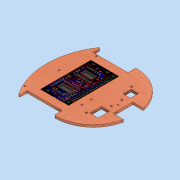
# Autodesk Inventor part: Version Raspberrry Pi Zero W
Saved by Autodesk Inventor 2022 (Build 260153000, 153)
## iProperties
Created: 2021-09-27
Part Number: Version Raspberrry Pi Zero W
Material: Madera (nogal)
Document SubType Name: Modeling
Designer: Julio R
Density: 0.55 g/cm^3
Appearance: Nogal - Natural pulido
Author: Julio R
Autodesk Inventor part; units mm, degrees
ref_plane "YZ Plane" through (0, 0, 0) normal (1, 0, 0) x (0, 1, 0)
ref_plane "XZ Plane" through (0, 0, 0) normal (0, 1, 0) x (-1, 0, 0)
ref_plane "XY Plane" through (0, 0, 0) normal (0, 0, 1) x (1, 0, 0)
sketch "Boceto2" plane through (0, 0, 0) normal (0, 1, 0) x (-1, 0, 0)
  circle A0 centre (-10.65, 0) radius 62.5
  line L0 (-44, 29.7) -> (-44, -29.3)
  line L1 (-41, -32.3) -> (-17, -32.3)
  line L2 (-14, -29.3) -> (-14, 29.7)
  line L3 (-17, 32.7) -> (-41, 32.7)
  circle A1 centre (-40.5, -28.8) radius 1.25
  line L4 (0, 6.809) -> (0, -6.809)
  line L5 (10.65, 0) -> (-10.65, 0) construction
  circle A2 centre (-17.5, -28.8) radius 1.25
  circle A3 centre (-40.5, 29.2) radius 1.25
  circle A4 centre (-17.5, 29.2) radius 1.25
  line L6 (7.5, -42.3) -> (-7, -42.3)
  line L7 (-7, -42.3) -> (-7, -25)
  line L8 (-7, -25) -> (7.5, -25)
  line L9 (7.5, -25) -> (7.5, -42.3)
  arc A5 (9.0958, -33.5419) -> (9.0958, -25.0441) centre (9, -29.293) ccw
  line L10 (9.0958, -33.5419) -> (7.5, -42.3)
  line L11 (9.0958, -25.0441) -> (7.5, -25.0441)
  arc A6 (9.5, -30.443) -> (9.5, -28.143) centre (9.5, -29.293) ccw
  line L12 (9.5, -30.443) -> (7.5, -30.443)
  line L13 (7.5, -30.443) -> (7.5, -28.143)
  line L14 (7.5, -28.143) -> (9.5, -28.143)
  line L15 (9.5, -28.143) -> (9.5, -30.443)
  arc A7 (-9.0958, -25.0441) -> (-9.0958, -33.5419) centre (-9, -29.293) ccw
  line L16 (-9.0958, -33.5419) -> (-7, -42.3)
  line L17 (-9.0958, -25.0441) -> (-7.5, -25.0441)
  arc A8 (-9.5, -28.143) -> (-9.5, -30.443) centre (-9.5, -29.293) ccw
  line L18 (-9.5, -30.443) -> (-7.5, -30.443)
  line L19 (-7.5, -30.443) -> (-7.5, -28.143)
  line L20 (-7.5, -28.143) -> (-9.5, -28.143)
  line L21 (-9.5, -28.143) -> (-9.5, -30.443)
  line L22 (7.5, 42.3) -> (-7, 42.3)
  line L23 (-7, 42.3) -> (-7, 25)
  line L24 (-7, 25) -> (7.5, 25)
  line L25 (7.5, 25) -> (7.5, 42.3)
  arc A9 (9.0958, 25.0441) -> (9.0958, 33.5419) centre (9, 29.293) ccw
  line L26 (9.0958, 33.5419) -> (7.5, 42.3)
  line L27 (9.0958, 25.0441) -> (7.5, 25.0441)
  arc A10 (9.5, 28.143) -> (9.5, 30.443) centre (9.5, 29.293) ccw
  line L28 (9.5, 30.443) -> (7.5, 30.443)
  line L29 (7.5, 30.443) -> (7.5, 28.143)
  line L30 (7.5, 28.143) -> (9.5, 28.143)
  line L31 (9.5, 28.143) -> (9.5, 30.443)
  line L32 (-9.0958, 25.0441) -> (-7.5, 25.0441)
  line L33 (-7.5, 28.143) -> (-9.5, 28.143)
  line L34 (-7.5, 30.443) -> (-7.5, 28.143)
  line L35 (-9.5, 28.143) -> (-9.5, 30.443)
  line L36 (-9.5, 30.443) -> (-7.5, 30.443)
  arc A11 (-9.5, 30.443) -> (-9.5, 28.143) centre (-9.5, 29.293) ccw
  line L37 (-9.0958, 33.5419) -> (-7, 42.3)
  arc A12 (-9.0958, 33.5419) -> (-9.0958, 25.0441) centre (-9, 29.293) ccw
  line L38 (10.3604, -4.25) -> (-9.8396, -4.25)
  line L39 (-9.8396, -4.25) -> (-9.8396, 4.25)
  line L40 (-9.8396, 4.25) -> (10.3604, 4.25)
  line L41 (10.3604, 4.25) -> (10.3604, -4.25)
  line L42 (35.3604, -42.3) -> (-56.6604, -42.3)
  line L43 (-56.6604, -42.3) -> (-56.6604, 42.3)
  line L44 (-56.6604, 42.3) -> (35.3604, 42.3)
  line L45 (35.3604, 42.3) -> (35.3604, -42.3)
  line L46 (-58.455, -12.75) -> (-68.455, -12.75)
  line L47 (-68.455, -12.75) -> (-68.455, 12.75)
  line L48 (-68.455, 12.75) -> (-58.455, 12.75)
  line L49 (-58.455, 12.75) -> (-58.455, -12.75)
  line L50 (22.5, 52.3) -> (-22.5, 52.3)
  line L51 (-22.5, 52.3) -> (-22.5, 42.3)
  line L52 (-22.5, 42.3) -> (22.5, 42.3)
  line L53 (22.5, 42.3) -> (22.5, 52.3)
  line L54 (22.5, -52.3) -> (-22.5, -52.3)
  line L55 (-22.5, -52.3) -> (-22.5, -42.3)
  line L56 (-22.5, -42.3) -> (22.5, -42.3)
  line L57 (22.5, -42.3) -> (22.5, -52.3)
  line L58 (22.5, 52.3) -> (23.5693, 52.3)
  line L59 (-22.5, 52.3) -> (-44.8693, 52.3)
  line L60 (22.5, -52.3) -> (23.5693, -52.3)
  line L61 (-22.5, -52.3) -> (-44.8693, -52.3)
  circle A13 centre (-49.1887, 5.7579) radius 1.15
  circle A14 centre (-49.1887, -7.7041) radius 1.15
  arc A15 (23.5693, -52.3) -> (23.5693, 52.3) centre (-52.609, 0) ccw
  line L62 (7.5, -18) -> (-7, -18)
  line L63 (-7, -18) -> (-7, -11.2)
  line L64 (-7, -11.2) -> (7.5, -11.2)
  line L65 (7.5, -11.2) -> (7.5, -18)
  line L66 (7.5, 11.5) -> (-7, 11.5)
  line L67 (-7, 11.5) -> (-7, 18.3)
  line L68 (-7, 18.3) -> (7.5, 18.3)
  line L69 (7.5, 18.3) -> (7.5, 11.5)
  circle A16 centre (24.1703, -0.4774) radius 1
  circle A17 centre (11.6311, 0) radius 1
  circle A18 centre (-11.1103, 0) radius 1
  arc A19 (-14, 29.7) -> (-17, 32.7) centre (-17, 29.7) ccw
  arc A20 (-17, -32.3) -> (-14, -29.3) centre (-17, -29.3) ccw
  arc A21 (-44, -29.3) -> (-41, -32.3) centre (-41, -29.3) ccw
  arc A22 (-41, 32.7) -> (-44, 29.7) centre (-41, 29.7) ccw
  line L70 (-14, 26.17) -> (-20.5456, 26.17)
  line L71 (-20.5456, 26.17) -> (-20.5456, -25.7515)
  line L72 (-20.5456, -25.7515) -> (-14, -25.7515)
  line L73 (-14, -25.7515) -> (-14, 26.17)
  line L74 (34.1703, -37.9774) -> (14.1703, -37.9774) construction
  line L75 (14.1703, -37.9774) -> (14.1703, 37.0226) construction
  line L76 (14.1703, 37.0226) -> (34.1703, 37.0226) construction
  line L77 (34.1703, 37.0226) -> (34.1703, -37.9774) construction
  circle A23 centre (28.6937, 39.0367) radius 1
  circle A24 centre (15.9449, -40.5329) radius 1
  circle A25 centre (-29, 23.17) radius 1
  circle A26 centre (-29, 11.2614) radius 1
  line L78 (-20.5456, 23.17) -> (-20.5456, 26.17)
  line L79 (-9.7082, -10.0259) -> (10.2918, -10.0259)
  line L80 (10.2918, -10.0259) -> (10.2918, 9.9741)
  line L81 (10.2918, 9.9741) -> (-9.7082, 9.9741)
  line L82 (-9.7082, 9.9741) -> (-9.7082, -10.0259)
  circle A27 centre (-51.964, -0.0259) radius 1
  point P0 (0, 0)
  point P1 (-14, -32.3)
  point P2 (-44, -32.3)
  point P3 (-14, 32.7)
  point P4 (-14, 0.2)
  point P5 (0, 0)
  point P6 (13.25, -29.293)
  point P7 (10.65, -29.293)
  point P8 (-13.25, -29.293)
  point P9 (-10.65, -29.293)
  point P10 (13.25, 29.293)
  point P11 (10.65, 29.293)
  point P12 (-10.65, 29.293)
  point P13 (-13.25, 29.293)
  point P14 (-16, 0)
  point P15 (10.3604, 0)
  point P16 (-58.455, 0)
  point P17 (-7.5, 36.9)
  point P18 (-7.5, 39.2)
  point P19 (-7.5, -39.2)
  point P20 (-7.5, -36.9)
  point P21 (7.5, -28.143)
  point P22 (7.5, -30.443)
  point P23 (-7, -42.3)
  point P24 (-56.6604, -42.3)
  point P25 (7.5, -42.3)
  point P26 (7.5, 42.3)
  point P27 (47.2734, 42.3)
  point P28 (-7, 42.3)
  point P29 (0, 52.3)
  point P30 (-22.5, -42.3)
  point P31 (22.5, -42.3)
  point P32 (22.5, 42.3)
  point P33 (-14, -25.7515)
  dimension "d128" = 125
  dimension "d52" = 65
  dimension "d53" = 30
  dimension "d56" = 3.5
  dimension "d57" = 3.5
  dimension "d60" = 23
  dimension "d63" = 58
  dimension "d78" = 14.5
  dimension "d79" = 17.3
  dimension "d81" = 1.5
  dimension "d82" = 4.25
  dimension "d83" = 1.15
  dimension "d84" = 2.3
  dimension "d86" = 2
  dimension "d88" = 7.5
  dimension "d92" = 20.2
  dimension "d93" = 8.5
  dimension "d94" = 10
  dimension "d95" = 25.5
  dimension "d108" = 10
  dimension "d113" = 45
  dimension "d114" = 13.462
  dimension "d116" = 2.3
  dimension "d119" = 2.3
  dimension "d120" = 14
  dimension "d127" = 25
  dimension "d133" = 10.65
  dimension "d134" = 42.3
  dimension "d135" = 1.5958
  dimension "d136" = 14.5
  dimension "d137" = 6.8
  dimension "d138" = 14.5
  dimension "d139" = 6.8
  dimension "d140" = 2
  dimension "d144" = 2
  dimension "d145" = 2
  dimension "d156" = 23
  dimension "d157" = 7
  dimension "d159" = 3
  dimension "d160" = 1.2707
  dimension "d161" = 1.2707
  dimension "d164" = 75
  dimension "d165" = 20
  dimension "d166" = 37.5
  dimension "d168" = 2
  dimension "d169" = 2
  dimension "d170" = 2
  dimension "d171" = 2
  dimension "d177" = 6.5457
  dimension "d178" = 10
  dimension "d179" = 51.9215
  dimension "d180" = 6.5485
  dimension "d181" = 11.9086
  dimension "d182" = 20
  dimension "d183" = 20
  dimension "d387" = 2
  constraints: 166 end point, 41 symmetric about line, 28 point on circle, 27 centre point, 24 parallel, 14 horizontal, 12 perpendicular, 12 point on line, 8 tangent, 6 midpoint, 5 vertical alignment, 4 coincident, 4 collinear, 4 horizontal alignment, 3 equal radius, 2 vertical, 21 other
  measures "d52" distance of point (-14, 32.7) point (-14, -32.3)
  measures "d53" distance of point (-14, -32.3) point (-44, -32.3)
  measures "d56" horizontal distance of A1.centre point (-44, -32.3)
  measures "d57" horizontal distance of point (-44, -32.3) A1.centre
  measures "d60" distance of A1.centre A2.centre
  measures "d63" distance of A1.centre A3.centre
  measures "d78" distance of L7.end L8.end
  measures "d79" distance of L6.end L7.end
  measures "d81" distance from line of L9 A5.centre
  measures "d82" radius of A5
  measures "d83" radius of A6
  measures "d84" distance between parallel lines of L14 L12
  measures "d86" distance from line of L13 A6.centre
  measures "d88" distance from line of point (0, 0) L9
  measures "d92" distance of L39.end L40.end
  measures "d93" distance of L38.end L39.end
  measures "d94" distance between parallel lines of L47 L49
  measures "d95" distance between parallel lines of L48 L46
  measures "d108" distance of L51.end L50.end
  measures "d113" distance between parallel lines of L51 L53
  measures "d114" distance of A14.centre A13.centre
  measures "d116" diameter of A13
  measures "d119" diameter of A14
  measures "d120" distance from line of L2 point (0, 0)
  measures "d127" distance between parallel lines of L45 L41
  measures "d133" distance of point (0, 0) point (-10.65, 0)
  measures "d134" distance from line of point (0, 0) L42
  measures "d135" distance from line of L9 L11.start
  measures "d136" distance of L63.end L64.end
  measures "d137" distance of L62.end L63.end
  measures "d138" distance of L67.end L68.end
  measures "d139" distance of L66.end L67.end
  measures "d140" diameter of A16
  measures "d144" diameter of A17
  measures "d145" diameter of A18
  measures "d156" diameter of L66 L5
  measures "d157" distance between parallel lines of L8 L62
  measures "d159" radius of A19
  measures "d160" distance from line of L41 A17.centre
  measures "d161" distance from line of L39 A18.centre
  measures "d164" distance between parallel lines of L76 L74
  measures "d165" distance between parallel lines of L75 L77
  measures "d166" distance from line of A16.centre L76
  measures "d168" diameter of A23
  measures "d169" diameter of A24
  measures "d170" diameter of A25
  measures "d171" diameter of A26
  measures "d177" distance between parallel lines of L73 L71
  measures "d178" distance between parallel lines of L1 L42
  measures "d179" distance between parallel lines of L70 L72
  measures "d180" distance between parallel lines of L1 L72
  measures "d181" distance of A26.centre A25.centre
  measures "d182" distance of L81.end L80.end
  measures "d183" distance of L80.end L79.end
  measures "d387" diameter of A27
extrude "Extrusión4" add sketch "Boceto2" along normal blind 3 contours A0 L45 A15 | L44 A15 A0 | L45 A15 L44 | A0 A15 L42 | L42 A15 L45 | L58 L50 L59 A0 | A15 L44 L53 L58 | A15 L45 L42 L10 A5 L11 L9 L8 L7 L43 L44 L23 L24 L25 L27 A9 L26 | A15 L45 | A0 L61 L54 L60 | L60 L57 L42 A15 | L59 L51 L44 A0 | L53 L44 L22 L51 L50 | A0 L42 L55 L61 | L54 L55 L42 L6 L57 | L43 A0 | L25 L24 L23 L22 | L26 A9 L27 L25 L30 A10 L28 | L6 L7 L8 L9 | L9 L12 A6 L14 L11 A5 L10 | L28 L31 L30 L25 | L9 L14 L15 L12 | A10 L31 | L15 A6 | A22 L3 A19 L2 L70 L71 L72 A20 L1 A21 L0 | L2 L72 L71 L70 | A1 | L40 L80 L38 L4 | L4 L38 L82 L40 | L40 L82 L81 L80 | L38 L80 L79 L82 | L82 L38 L39 L40 | L40 L41 L38 L80 | A2 | A3 | A4 | L21 A8 | L20 L19 L18 L21 | L33 L35 L36 L34 | A11 L35 | L46 L47 L48 L49 | A13 | A14 | L62 L63 L64 L65 | L66 L67 L68 L69 | A16 | A17 | A18 | A23 | A24 | A25 | A26 | A27
extrude "Extrusión9" cut sketch "Boceto2" along normal blind 3 contours A0 L45 A15 | L44 A15 A0 | L45 A15 L44 | A0 A15 L42 | L42 A15 L45 | L58 L50 L59 A0 | A0 L61 L54 L60 | L53 L44 L22 L51 L50 | L54 L55 L42 L6 L57 | L28 L31 L30 L25 | L9 L14 L15 L12 | A10 L31 | L15 A6 | A1 | L40 L80 L38 L4 | L4 L38 L82 L40 | L82 L38 L39 L40 | L40 L41 L38 L80 | A2 | A3 | A4 | L21 A8 | L20 L19 L18 L21 | L33 L35 L36 L34 | A11 L35 | L46 L47 L48 L49 | A13 | A14 | L62 L63 L64 L65 | L66 L67 L68 L69 | A17 | A18
fillet "Empalme6" radius 1 10 edges at (-23.5693, 1.5, 52.3) (-22.5, 1.5, 52.3) (-23.5693, 1.5, -52.3) (-22.5, 1.5, -52.3) (22.5, 1.5, -52.3) (22.5, 1.5, 52.3) (22.5, 1.5, -42.3) (-22.5, 1.5, -42.3) (-22.5, 1.5, 42.3) (22.5, 1.5, 42.3)
fillet "Empalme7" radius 49 2 edges at (44.8693, 1.5, 52.3) (44.8693, 1.5, -52.3)
extrude "Extrusión11" cut sketch "Boceto2" along normal blind 3 contours A2 | A4 | A16
extrude "Extrusión12" cut sketch "Boceto2" along normal blind 3 contours L2 L72 L71 L70 | A23 | A24 | A25 | A26
sketch "Boceto3" plane through (0, 3, 0) normal (0, 1, 0) x (1, 0, 0)
  line L0 (20.8865, 32.3) -> (20.8865, -32.7)
  line L1 (20.8865, -32.7) -> (-14.1135, -32.7)
  line L2 (-14.1135, -32.7) -> (-14.1135, 32.3)
  line L3 (20.8865, 32.3) -> (-14.1135, 32.3)
  circle A0 centre (17.5, 28.8) radius 1.25 projected
  circle A1 centre (17.5, -29.2) radius 1.25 projected
  circle A2 centre (29, -11.2614) radius 1 projected
  circle A3 centre (29, -23.17) radius 1 projected
  circle A4 centre (-28.6937, -39.0367) radius 1 projected
  line L4 (20.5456, 25.7515) -> (20.5456, -26.17) projected
  line L5 (20.5456, -26.17) -> (14, -26.17) projected
  line L6 (14, -26.17) -> (14, 25.7515) projected
  line L7 (14, 25.7515) -> (20.5456, 25.7515) projected
  circle A5 centre (-15.9449, 40.5329) radius 1 projected
  circle A6 centre (-24.1703, 0.4774) radius 1 projected
  arc A7 (71.254, 15.2778) -> (23.7405, 52.3) centre (23.7405, 3.3) ccw projected
  line L8 (23.7405, 52.3) -> (23.5, 52.3) projected
  arc A8 (23.5, 52.3) -> (22.5, 51.3) centre (23.5, 51.3) ccw projected
  line L9 (22.5, 51.3) -> (22.5, 43.3) projected
  arc A9 (21.5, 42.3) -> (22.5, 43.3) centre (21.5, 43.3) ccw projected
  line L10 (21.5, 42.3) -> (-21.5, 42.3) projected
  arc A10 (-22.5, 43.3) -> (-21.5, 42.3) centre (-21.5, 43.3) ccw projected
  line L11 (-22.5, 43.3) -> (-22.5, 50.6166) projected
  arc A11 (-22.5, 50.6166) -> (-24.3327, 51.1703) centre (-23.5, 50.6166) ccw projected
  arc A12 (-24.3327, 51.1703) -> (-24.3327, -51.1703) centre (52.609, 0) ccw projected
  arc A13 (-24.3327, -51.1703) -> (-22.5, -50.6166) centre (-23.5, -50.6166) ccw projected
  line L12 (-22.5, -50.6166) -> (-22.5, -43.3) projected
  arc A14 (-21.5, -42.3) -> (-22.5, -43.3) centre (-21.5, -43.3) ccw projected
  line L13 (-21.5, -42.3) -> (21.5, -42.3) projected
  arc A15 (22.5, -43.3) -> (21.5, -42.3) centre (21.5, -43.3) ccw projected
  line L14 (22.5, -43.3) -> (22.5, -51.3) projected
  arc A16 (22.5, -51.3) -> (23.5, -52.3) centre (23.5, -51.3) ccw projected
  line L15 (23.5, -52.3) -> (23.7405, -52.3) projected
  arc A17 (23.7405, -52.3) -> (71.254, -15.2778) centre (23.7405, -3.3) ccw projected
  arc A18 (71.254, -15.2778) -> (71.254, 15.2778) centre (10.65, 0) ccw projected
  line L16 (-7.5, 11.2) -> (-7.5, 18) projected
  line L17 (-7.5, 18) -> (7, 18) projected
  line L18 (7, 18) -> (7, 11.2) projected
  line L19 (7, 11.2) -> (-7.5, 11.2) projected
  circle A19 centre (40.5, -29.2) radius 1.25 projected
  arc A20 (-9.5, 30.443) -> (-9.5, 28.143) centre (-9.5, 29.293) ccw projected
  line L20 (-9.5, 30.443) -> (-7.5, 30.443) projected
  line L21 (-7.5, 30.443) -> (-7.5, 28.143) projected
  line L22 (-7.5, 28.143) -> (-9.5, 28.143) projected
  line L23 (58.455, -12.75) -> (58.455, 12.75) projected
  line L24 (58.455, 12.75) -> (68.455, 12.75) projected
  line L25 (68.455, 12.75) -> (68.455, -12.75) projected
  line L26 (68.455, -12.75) -> (58.455, -12.75) projected
  circle A21 centre (49.1887, 7.7041) radius 1.15 projected
  line L27 (-7.5, -30.443) -> (-9.5, -30.443) projected
  arc A22 (-9.5, -28.143) -> (-9.5, -30.443) centre (-9.5, -29.293) ccw projected
  line L28 (-9.5, -28.143) -> (-7.5, -28.143) projected
  line L29 (-7.5, -28.143) -> (-7.5, -30.443) projected
  circle A23 centre (17.5, 28.8) radius 1.25 projected
  line L30 (-7.5, -18.3) -> (-7.5, -11.5) projected
  line L31 (-7.5, -11.5) -> (7, -11.5) projected
  line L32 (7, -11.5) -> (7, -18.3) projected
  line L33 (7, -18.3) -> (-7.5, -18.3) projected
  circle A24 centre (11.1103, 0) radius 1 projected
  circle A25 centre (17.5, -29.2) radius 1.25 projected
  line L34 (7.5, 30.443) -> (9.5, 30.443) projected
  arc A26 (9.5, 28.143) -> (9.5, 30.443) centre (9.5, 29.293) ccw projected
  line L35 (9.5, 28.143) -> (7.5, 28.143) projected
  line L36 (7.5, 28.143) -> (7.5, 30.443) projected
  circle A27 centre (49.1887, -5.7579) radius 1.15 projected
  arc A28 (9.5, -30.443) -> (9.5, -28.143) centre (9.5, -29.293) ccw projected
  line L37 (9.5, -30.443) -> (7.5, -30.443) projected
  line L38 (7.5, -30.443) -> (7.5, -28.143) projected
  line L39 (7.5, -28.143) -> (9.5, -28.143) projected
  circle A29 centre (40.5, 28.8) radius 1.25 projected
  line L40 (-10.3604, -4.25) -> (-10.3604, 4.25) projected
  line L41 (-10.3604, 4.25) -> (9.8396, 4.25) projected
  line L42 (9.8396, 4.25) -> (9.8396, -4.25) projected
  line L43 (9.8396, -4.25) -> (-10.3604, -4.25) projected
  circle A30 centre (-11.6311, 0) radius 1 projected
  line L44 (-15.606, -33.2472) -> (-15.606, 32.7528) construction
  line L45 (-15.606, 32.7528) -> (21.4726, 32.7528) construction
  line L46 (21.4726, 32.7528) -> (21.4726, -33.2472) construction
  line L47 (21.4726, -33.2472) -> (-15.606, -33.2472) construction
  line L48 (-9.0297, -25.5314) -> (9.3868, -25.5314)
  line L49 (9.3868, -25.5314) -> (9.3868, -22.2663)
  line L50 (9.3868, -22.2663) -> (-9.0297, -22.2663)
  line L51 (-9.0297, -22.2663) -> (-9.0297, -25.5314)
  line L52 (-9.0297, 20.6397) -> (7.7218, 20.6397)
  line L53 (7.7218, 20.6397) -> (7.7218, 24.3886)
  line L54 (7.7218, 24.3886) -> (-9.0297, 24.3886)
  line L55 (-9.0297, 24.3886) -> (-9.0297, 20.6397)
  line L56 (14, -26.17) -> (14, 25.7515) projected
  line L57 (9.3868, -32.0744) -> (14, -32.0744)
  line L58 (14, -32.0744) -> (14, -12.5)
  line L59 (14, -12.5) -> (9.3868, -12.5)
  line L60 (9.3868, -12.5) -> (9.3868, -32.0744)
  line L61 (-13.8057, -19.8238) -> (-9.4895, -19.8238)
  line L62 (-9.4895, -19.8238) -> (-9.4895, -4.6772)
  line L63 (-9.4895, -4.6772) -> (-13.8057, -4.6772)
  line L64 (-13.8057, -4.6772) -> (-13.8057, -19.8238)
  line L65 (-13.3666, 8.9365) -> (-9.4895, 8.9365)
  line L66 (-9.4895, 8.9365) -> (-9.4895, 15.1891)
  line L67 (-9.4895, 15.1891) -> (-13.3666, 15.1891)
  line L68 (-13.3666, 15.1891) -> (-13.3666, 8.9365)
  line L69 (-9.4895, -9.55) -> (10.9255, -9.55)
  line L70 (10.9255, -9.55) -> (10.9255, -6.55)
  line L71 (10.9255, -6.55) -> (-9.4895, -6.55)
  line L72 (-9.4895, -6.55) -> (-9.4895, -9.55)
  line L73 (-9.4895, 5.75) -> (10.9255, 5.75)
  line L74 (10.9255, 5.75) -> (10.9255, 8.75)
  line L75 (10.9255, 8.75) -> (-9.4895, 8.75)
  line L76 (-9.4895, 8.75) -> (-9.4895, 5.75)
  line L77 (9.3868, -12.5) -> (7.3247, -12.5)
  line L78 (7.3247, -12.5) -> (7.3247, -21.1057)
  line L79 (7.3247, -21.1057) -> (9.3868, -21.1057)
  line L80 (9.3868, -21.1057) -> (9.3868, -12.5)
  line L81 (52.609, 15.5566) -> (43.1767, 15.5566)
  line L82 (43.1767, 15.5566) -> (43.1767, 25.7515)
  line L83 (43.1767, 25.7515) -> (52.609, 25.7515)
  line L84 (52.609, 25.7515) -> (52.609, 15.5566)
  line L85 (53.8576, -27.3152) -> (43.1767, -27.3152)
  line L86 (43.1767, -27.3152) -> (43.1767, -12.5)
  line L87 (43.1767, -12.5) -> (53.8576, -12.5)
  line L88 (53.8576, -12.5) -> (53.8576, -27.3152)
  line L89 (68.455, 12.75) -> (71.8357, 12.75)
  line L90 (68.455, -12.75) -> (58.455, -12.75) projected
  line L91 (68.455, -12.75) -> (71.8357, -12.75)
  point P0 (0, 0)
  dimension "d184" = 35
  dimension "d185" = 65
  dimension "d186" = 3.5
  dimension "d187" = 3.5
  dimension "d188" = 6.8
  dimension "d189" = 6.6135
  dimension "d193" = 2.257
  dimension "d194" = 1.857
  dimension "d195" = 8.5
  dimension "d196" = 14.5
  dimension "d197" = 6.8
  dimension "d198" = 14.5
  dimension "d200" = 6.6135
  dimension "d202" = 14.4
  dimension "d203" = 13.8865
  dimension "d204" = 43.9
  dimension "d205" = 31.247
  dimension "d206" = 28.45
  dimension "d207" = 2
  dimension "d209" = 13.3865
  dimension "d210" = 13.3865
  dimension "d211" = 15
  dimension "d212" = 13.3865
  dimension "d213" = 28.3865
  dimension "d331" = 66
  dimension "d377" = 3
  dimension "d378" = 3
  dimension "d381" = 1.5
  dimension "d382" = 2.3
  constraints: 92 end point, 20 parallel, 12 horizontal, 11 perpendicular, 7 point on line, 3 vertical, 2 point on circle, 1 collinear, 2 other
  measures "d184" distance of L0.start L2.end
  measures "d185" distance of L1.end L2.end
  measures "d186" distance from line of L3 A0.centre
  measures "d187" distance from line of L1 A1.centre
  measures "d188" distance between parallel lines of L19 L17
  measures "d189" distance between parallel lines of L2 L16
  measures "d193" distance between parallel lines of L1 L37
  measures "d194" distance between parallel lines of L3 L34
  measures "d195" distance between parallel lines of L43 L41
  measures "d196" distance between parallel lines of L16 L18
  measures "d197" distance between parallel lines of L33 L31
  measures "d198" distance between parallel lines of L30 L32
  measures "d200" distance between parallel lines of L2 L30
  measures "d202" vertical distance of L0.end L32.end
  measures "d203" horizontal distance of L0.end L32.end
  measures "d204" vertical distance of L0.end L18.end
  measures "d205" horizontal distance of L0.end L40.start
  measures "d206" vertical distance of L0.end L40.start
  measures "d207" distance from line of A26.centre L36
  measures "d209" horizontal distance of L0.start L34.start
  measures "d210" distance between parallel lines of L0 L38
  measures "d211" distance between parallel lines of L38 L29
  measures "d212" distance from line of L0.start L36
  measures "d213" distance between parallel lines of L0 L21
  measures "d331" distance of L44.start L44.end
  measures "d377" distance between parallel lines of L73 L75
  measures "d378" distance between parallel lines of L69 L71
  measures "d381" distance between parallel lines of L73 L41
  measures "d382" distance between parallel lines of L43 L71
extrude "Extrusión13" cut sketch "Boceto3" against normal blind 3 contours A18 L91 L25 L89 | L62 L71 L70 L69 | L76 L75 L74 L73 | L81 L82 L83 L84 | L85 L86 L87 L88
extrude "Extrusión14" cut sketch "Boceto2" along normal blind 3 contours A27
sketch "Boceto4" plane through (0, 3, 0) normal (0, 1, 0) x (1, 0, 0)
  line L0 (-15.5027, -32.8633) -> (-15.5027, 32.6151) construction
  line L1 (-15.5027, 32.6151) -> (21.2829, 32.6151) construction
  line L2 (21.2829, 32.6151) -> (21.2829, -32.8633) construction
  line L3 (21.2829, -32.8633) -> (-15.5027, -32.8633) construction
  point P0 (0, 0)
  constraints: 1 vertical, 2 other
